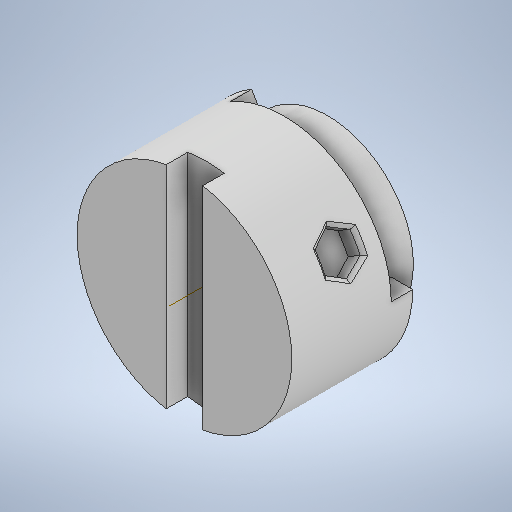
# Autodesk Inventor part: ToolMount
Saved by Autodesk Inventor 2025.3 (Build 293356030, 356C)
## iProperties
Created: 2025-10-10
Part Number: ToolMount
Material: Generic
Document SubType Name: Modeling
Designer: tvoko
Density: 1 g/cm^3
Appearance: Default
Author: tvoko
Autodesk Inventor part; units mm, degrees
ref_plane "YZ Plane" through (0, 0, 0) normal (1, 0, 0) x (0, 1, 0)
ref_plane "XZ Plane" through (0, 0, 0) normal (0, 1, 0) x (-1, 0, 0)
ref_plane "XY Plane" through (0, 0, 0) normal (0, 0, 1) x (1, 0, 0)
sketch "Sketch2" plane through (0, 0, 0) normal (0, 0, 1) x (1, 0, 0)
  circle A0 centre (0, 0) radius 15
  line L0 (-2.55, 0) -> (2.55, 0) construction
  line L1 (-2.55, 14.7817) -> (-2.55, -14.7817)
  line L2 (2.55, 14.7817) -> (2.55, -14.7817)
  dimension "d0" = 5.1
  dimension "d1" = 30
  constraints: 6 end point, 4 point on circle, 3 midpoint, 2 coincident, 1 centre point, 1 horizontal
  measures "d0" distance between parallel lines of L2 L1
  measures "d1" diameter of A0
extrude "Extrusion1" add sketch "Sketch2" against normal blind 20
extrude "Extrusion2" cut sketch "Sketch2" against normal blind 3 contours L2 A0 L1
sketch "Sketch4" plane through (0, 0, -20) normal (0, 0, -1) x (-1, 0, 0)
  circle A0 centre (0, 0) radius 15 projected
  line L0 (7.5, 12.9904) -> (-7.5, -12.9904)
  line L1 (15, 0) -> (-15, 0)
  line L2 (0, 15) -> (0, -15) construction
  circle A1 centre (0, 0) radius 12
  point P0 (-6, -10.3923)
  point P1 (12, 0)
  point P2 (-12, 0)
  point P3 (6, 10.3923)
  dimension "d9" = 90
  dimension "d10" = 60
  dimension "d11" = 3
  constraints: 6 end point, 5 point on circle, 4 midpoint, 1 centre point, 1 vertical
  measures "d9" angle of L1 L2
  measures "d10" angle of L0 L1
  measures "d11" radial gap between concentric circles of A0 A1
extrude "Extrusion4" cut sketch "Sketch4" against normal blind 6.1 contours A0 L0 A1 L1 | L0 A1 L1 A0 picked at (-5.934, -12.5842) picked at (5.934, 12.5842)
extrude "Extrusion5" cut sketch "Sketch4" against normal blind 3.1 contours L1 A1 L0 A0 | A0 L1 A1 L0 picked at (7.8456, 11.51) picked at (-7.8456, -11.51)
ref_plane "Work Plane1" through (0, 0, -20) normal (-0.5, 0.8660254, 0) x (0, 0, 1)
sketch "Sketch5" plane through (0, 0, -20) normal (-0.5, 0.8660254, 0) x (0, 0, 1)
  line L0 (17, -9.5992) -> (20, -9.5992) projected
  line L1 (20, 5.1825) -> (20, -9.5992) projected
  line L2 (20, 5.1825) -> (17, 5.1825) projected
  line L3 (17, 5.1825) -> (17, 9.5992) projected
  line L4 (17, 9.5992) -> (20, 9.5992) projected
  line L5 (20, -5.1825) -> (20, 9.5992) projected
  line L6 (20, -5.1825) -> (17, -5.1825) projected
  line L7 (17, -5.1825) -> (17, -9.5992) projected
  line L8 (3.1, 0) -> (3.1, 12.9904) projected
  line L9 (3.1, 12.9904) -> (6.1, 12.9904) projected
  line L10 (6.1, 12.9904) -> (6.1, 0) projected
  line L11 (6.1, 0) -> (3.1, 0) projected
  line L12 (3.1, 0) -> (3.1, -12.9904) projected
  line L13 (3.1, -12.9904) -> (6.1, -12.9904) projected
  line L14 (6.1, -12.9904) -> (6.1, 0) projected
  line L15 (6.1, 0) -> (3.1, 0) projected
  line L16 (20, 2.9445) -> (17, 2.9445) projected
  line L17 (17, 2.9445) -> (17, -2.9445) projected
  line L18 (17, -2.9445) -> (20, -2.9445) projected
  line L19 (20, -2.9445) -> (20, -15) projected
  line L20 (20, -15) -> (6.1, -15) projected
  line L21 (6.1, -15) -> (6.1, -12) projected
  line L22 (6.1, -12) -> (0, -12) projected
  line L23 (0, -12) -> (0, 12) projected
  line L24 (0, 12) -> (6.1, 12) projected
  line L25 (6.1, 12) -> (6.1, 15) projected
  line L26 (6.1, 15) -> (20, 15) projected
  line L27 (20, 15) -> (20, 2.9445) projected
  point P0 (20, 0)
ref_plane "Work Plane2" through (12.9904, 7.5, -13.9) normal (0.8660254, 0.5, 0) x (-0.5, 0.8660254, 0)
sketch "Sketch6" plane through (12.9904, 7.5, -13.9) normal (0.8660254, 0.5, 0) x (-0.5, 0.8660254, 0)
  line L0 (-1.4145, 7.45) -> (1.4145, 7.45)
  line L1 (1.4145, 7.45) -> (2.829, 5)
  line L2 (2.829, 5) -> (1.4145, 2.55)
  line L3 (1.4145, 2.55) -> (-1.4145, 2.55)
  line L4 (-1.4145, 2.55) -> (-2.829, 5)
  line L5 (-2.829, 5) -> (-1.4145, 7.45)
  line L6 (15, 0) -> (-7.5, 0) projected
  line L7 (0, 0) -> (0, 13.9) construction
  point P0 (0, 5)
  dimension "d17" = 4.9
  dimension "d18" = 5
  constraints: 12 end point, 1 parallel, 1 point on line, 13 other
  measures "d17" distance between parallel lines of L3 L0
  measures "d18" distance from line of L6 point (0, 5)
extrude "Extrusion6" cut sketch "Sketch6" against normal blind 2.5
chamfer "Chamfer1" distance 0.5 angle 45 6 edges at (13.9216, 5.5848, -7.6792) (12.9904, 7.5, -6.45) (11.7974, 9.264, -7.6792) (11.7974, 9.264, -10.1208) (12.9904, 7.5, -11.35) (13.9216, 5.5848, -10.1208)
body "Solid1"
